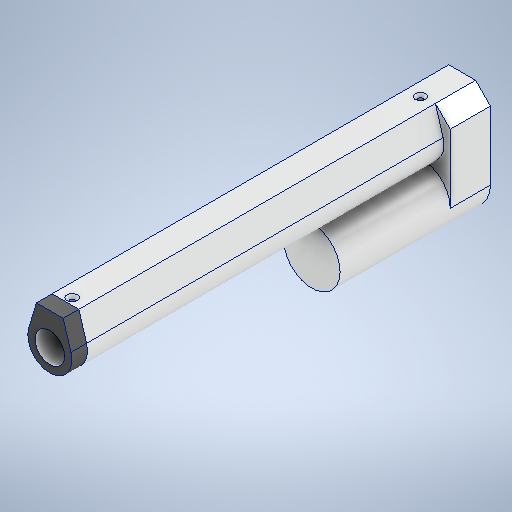
# Autodesk Inventor part: Linear Motor (T-Frame)
Saved by Autodesk Inventor 2026.1 (Build 301233000, 233)
## iProperties
Created: 2026-04-11
Part Number: Linear Motor (T-Frame)
Material: Aluminum 6061
Document SubType Name: Modeling
Designer: chanh
Density: 2.7 g/cm^3
Appearance: Aluminum - Flat
Author: chanh
Autodesk Inventor part; units mm, degrees
ref_plane "YZ Plane" through (0, 0, 0) normal (1, 0, 0) x (0, 1, 0)
ref_plane "XZ Plane" through (0, 0, 0) normal (0, 1, 0) x (-1, 0, 0)
ref_plane "XY Plane" through (0, 0, 0) normal (0, 0, 1) x (1, 0, 0)
sketch "Sketch1" plane through (0, 0, 0) normal (0, 0, 1) x (1, 0, 0)
  circle A0 centre (0, 0) radius 14.8
  line L0 (-9, 21.5) -> (9, 21.5)
  line L1 (-9, 21.5) -> (-19, 11.5)
  line L2 (-19, 11.5) -> (-19, -34.776357)
  circle A1 centre (0, -34.5) radius 19
  line L3 (0, 21.5) -> (0, -34.5) construction
  line L4 (9, 21.5) -> (19, 11.5)
  line L5 (19, 11.5) -> (19, -34.776357)
  point P0 (-19, -34.5)
  point P1 (19, -34.5)
  dimension "d0" = 29.6
  dimension "d1" = 18
  dimension "d2" = 21.5
  dimension "d3" = 38
  dimension "d4" = 56
  dimension "d5" = 45
  constraints: 12 end point, 2 centre point, 2 symmetric about line, 2 vertical, 2 vertical alignment, 1 coincident, 1 horizontal, 1 midpoint, 1 tangent
  measures "d0" diameter of A0
  measures "d1" distance of L0.start L0.end
  measures "d2" distance of point (0, 0) L3.start
  measures "d3" diameter of A1
  measures "d4" distance from line of L3.end L0
  measures "d5" angle of L0 L1
sketch "Sketch1 outline for Extrusion1" plane through (0, 0, 0) normal (0, 0, 1) x (1, 0, 0)
  line L0 (19, 11.5) -> (9, 21.5)
  line L1 (19, -34.5) -> (19, 11.5)
  arc A0 (-19, -34.5) -> (19, -34.5) centre (0, -34.5) ccw
  line L2 (-19, 11.5) -> (-19, -34.5)
  line L3 (-9, 21.5) -> (-19, 11.5)
  line L4 (9, 21.5) -> (-9, 21.5)
extrude "Extrusion1" add sketch "Sketch1 outline for Extrusion1" along normal blind 27
sketch "Sketch2" plane through (0, 0, 27) normal (0, 0, 1) x (1, 0, 0)
  line L0 (9, 21.5) -> (-9, 21.5)
  circle A0 centre (0, 0) radius 14.8
  line L1 (-9, 21.5) -> (-14.175455, 4.253996)
  line L2 (9, 21.5) -> (14.175455, 4.253996)
  line L3 (9, 21.5) -> (-9, 21.5)
  line L4 (-9, 21.5) -> (9, 21.5)
  dimension "d8" = 29.6
  constraints: 8 end point, 2 point on circle, 2 tangent, 1 centre point, 1 coincident, 1 collinear
  measures "d8" diameter of A0
extrude "Extrusion2" add sketch "Sketch2" along normal blind 250
sketch "Sketch3" plane through (0, 0, 27) normal (0, 0, 1) x (1, 0, 0)
  arc A0 (-19, -34.5) -> (19, -34.5) centre (0, -34.5) ccw projected
  circle A1 centre (0, -34.5) radius 19
  point P0 (0, 0)
  point P1 (19, -34.5)
  point P2 (-19, -34.5)
  constraints: 1 centre point, 1 coincident, 1 concentric
extrude "Extrusion3" add sketch "Sketch3" along normal blind 74
sketch "Sketch4" plane through (-9, 21.5, 0) normal (0, 1, 0) x (1, 0, 0)
  line L0 (18, 0) -> (0, 0) projected
  line L1 (0, 0) -> (0, -27) projected
  line L2 (0, -27) -> (0, -277) projected
  line L3 (18, -277) -> (0, -277) projected
  line L4 (18, -27) -> (18, -277) projected
  line L5 (18, 0) -> (18, -27) projected
  line L6 (-16, -266.5) -> (34, -266.5)
  point P0 (9, 0)
  point P1 (9, -266.5)
  point P2 (9, -277)
  dimension "d13" = 50
  dimension "d14" = 10.5
  constraints: 2 end point, 2 midpoint, 1 horizontal, 1 vertical alignment
  measures "d13" distance of L6.start L6.end
  measures "d14" distance between parallel lines of L6 L3
split_face "Split1"
sketch "Sketch5" plane through (0, 0, 277) normal (0, 0, 1) x (1, 0, 0)
  circle A0 centre (0, 0) radius 10
  dimension "d15" = 20
  constraints: 1 centre point, 1 coincident
  measures "d15" diameter of A0
extrude "Extrusion4" cut sketch "Sketch5" against normal blind 427
sketch "Sketch6" plane through (-9, 21.5, 0) normal (0, 1, 0) x (1, 0, 0)
  line L0 (18, -266.5) -> (0, -266.5) projected
  line L1 (18, -27) -> (18, -266.5) projected
  line L2 (18, 0) -> (18, -27) projected
  line L3 (18, 0) -> (0, 0) projected
  line L4 (0, 0) -> (0, -27) projected
  line L5 (0, -27) -> (0, -266.5) projected
  line L6 (18, -266.5) -> (0, -266.5) projected
  line L7 (0, -266.5) -> (0, -277) projected
  line L8 (18, -277) -> (0, -277) projected
  line L9 (18, -266.5) -> (18, -277) projected
  point P0 (9, 0)
  point P1 (9, -262)
  point P2 (9, -28)
  point P3 (9, 0)
  point P4 (9, -277)
  dimension "d18" = 28
  dimension "d19" = 15
  constraints: 2 midpoint, 2 vertical alignment
  measures "d18" distance from line of L3 point (9, -28)
  measures "d19" distance from line of L8 point (9, -262)
hole "Hole1" at (0, 21.5, 262) at (0, 21.5, 28) direction (0, -1, 0) diameter 3.242 depth 8 countersink diameter 7 countersink angle 90 thread size "M4x0.7" class "6H" standard "ISO Metric profile"
body "Solid1"
